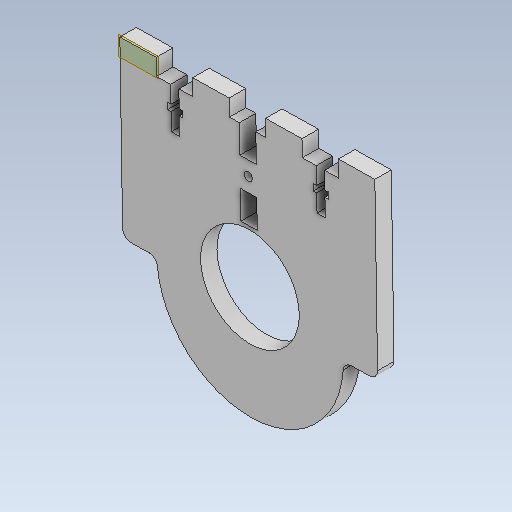
# Autodesk Inventor part: Деталь1
Saved by Autodesk Inventor 2021.1 (Build 251245010, 245A)
## iProperties
Created: 2023-03-16
Part Number: Деталь1
Material: Типовые
Document SubType Name: Modeling
Designer: User
Density: 1 g/cm^3
Appearance: По умолчанию
Author: User
Autodesk Inventor part; units mm, degrees
ref_plane "YZ Plane" through (0, 0, 0) normal (1, 0, 0) x (0, 1, 0)
ref_plane "XZ Plane" through (0, 0, 0) normal (0, 1, 0) x (-1, 0, 0)
ref_plane "XY Plane" through (0, 0, 0) normal (0, 0, 1) x (1, 0, 0)
ref_plane "РабПлоскость1" through (67.2056, 19.9956, 394.3851) normal (0, 0, -1) x (-0.9999, -0.0165, 0)
sketch "Эскиз1" plane through (67.2056, 19.9956, 394.3851) normal (0, 0, -1) x (-0.9999, -0.0165, 0)
  line L0 (-9.6218, -57.1442) -> (-3, -57.1442) projected
  arc A0 (-9.6218, -57.1442) -> (-12.6119, -59.9009) centre (-9.6218, -60.1442) ccw projected
  arc A1 (-3, -57.1442) -> (0, -54.1442) centre (-3, -54.1442) ccw projected
  line L1 (0, -54.1442) -> (0, 5.8558) projected
  line L2 (0, 5.8558) -> (-13.2857, 5.8558) projected
  line L3 (-13.2857, -0.1442) -> (-13.2857, 5.8558) projected
  line L4 (-13.2857, -0.1442) -> (-26.5714, -0.1442)
  line L5 (-26.5714, -0.1442) -> (-26.5714, 5.8558)
  line L6 (-26.5714, 5.8558) -> (-39.8571, 5.8558) projected
  line L7 (-39.8571, -0.1442) -> (-39.8571, 5.8558) projected
  line L8 (-39.8571, -0.1442) -> (-53.1429, -0.1442)
  line L9 (-53.1429, -0.1442) -> (-53.1429, 5.8558)
  line L10 (-53.1429, 5.8558) -> (-66.4286, 5.8558) projected
  line L11 (-66.4286, -0.1442) -> (-66.4286, 5.8558) projected
  line L12 (-66.4286, -0.1442) -> (-79.7143, -0.1442)
  line L13 (-79.7143, -0.1442) -> (-79.7143, 5.8558)
  line L14 (-79.7143, 5.8558) -> (-93, 5.8558) projected
  line L15 (-93, 5.8558) -> (-93, -54.1442) projected
  arc A2 (-93, -54.1442) -> (-90, -57.1442) centre (-90, -54.1442) ccw projected
  line L16 (-90, -57.1442) -> (-83.3782, -57.1442) projected
  arc A3 (-80.3881, -59.9009) -> (-83.3782, -57.1442) centre (-83.3782, -60.1442) ccw projected
  arc A4 (-80.3881, -59.9009) -> (-12.6119, -59.9009) centre (-46.5, -57.1442) ccw projected
  circle A5 centre (-46.5, -50.1442) radius 18
  line L17 (-74.5714, -0.1442) -> (-79.7143, -0.1442) projected
  line L18 (-21.4286, -0.1442) -> (-26.5714, -0.1442) projected
  line L19 (-49.5, -0.1442) -> (-53.1429, -0.1442) projected
  circle A6 centre (-46.5, -50.1442) radius 18 construction
  point P0 (67.5262, -18.8845)
  dimension "d0" = 6
  constraints: 12 end point, 1 centre point, 1 coincident, 1 concentric
  measures "d0" distance of L3.start L2.end
extrude "Выдавливание1" add sketch "Эскиз1" along normal blind 6
sketch "Эскиз2" plane through (67.2056, 19.9956, 388.3851) normal (0, 0, -1) x (-0.9999, -0.0165, 0)
  circle A0 centre (-46.5, -15.5) radius 1.5 projected
  line L0 (-49.5, -10.3334) -> (-49.5, -0.1442) construction
  line L1 (-43.5, -0.1442) -> (-43.5, -10.3334) construction
  line L2 (-43.5, -20.6667) -> (-43.5, -31) construction
  line L3 (-49.5, -31) -> (-49.5, -20.6667) construction
  line L4 (-49.5, -31) -> (-43.5, -31)
  line L5 (-43.5, -31) -> (-43.5, -20.6667)
  line L6 (-43.5, -20.6667) -> (-49.5, -20.6667)
  line L7 (-49.5, -20.6667) -> (-49.5, -31)
  line L8 (-49.5, -10.3334) -> (-43.5, -10.3334)
  line L9 (-43.5, -10.3334) -> (-43.5, -0.1442)
  line L10 (-43.5, -0.1442) -> (-49.5, -0.1442)
  line L11 (-49.5, -0.1442) -> (-49.5, -10.3334)
  line L12 (-17.1786, -8.65) -> (-17.1786, -6.35)
  line L13 (-17.1786, -6.35) -> (-18.4286, -6.35)
  line L14 (-18.4286, -6.35) -> (-18.4286, -0.1442)
  line L15 (-21.4286, -0.1442) -> (-21.4286, -6.35)
  line L16 (-21.4286, -6.35) -> (-22.6786, -6.35)
  line L17 (-22.6786, -6.35) -> (-22.6786, -8.65)
  line L18 (-22.6786, -8.65) -> (-21.4286, -8.65)
  line L19 (-21.4286, -8.65) -> (-21.4286, -15)
  line L20 (-21.4286, -15) -> (-18.4286, -15)
  line L21 (-18.4286, -15) -> (-18.4286, -8.65)
  line L22 (-18.4286, -8.65) -> (-17.1786, -8.65)
  line L23 (-21.4286, -0.1442) -> (-18.4286, -0.1442)
  line L24 (-46.5, -10.3334) -> (-46.5, -0.1442) construction
  line L25 (-75.8214, -8.65) -> (-75.8214, -6.35)
  line L26 (-75.8214, -6.35) -> (-74.5714, -6.35)
  line L27 (-74.5714, -6.35) -> (-74.5714, -0.1442)
  line L28 (-71.5714, -0.1442) -> (-71.5714, -6.35)
  line L29 (-71.5714, -6.35) -> (-70.3214, -6.35)
  line L30 (-70.3214, -6.35) -> (-70.3214, -8.65)
  line L31 (-70.3214, -8.65) -> (-71.5714, -8.65)
  line L32 (-71.5714, -8.65) -> (-71.5714, -15)
  line L33 (-71.5714, -15) -> (-74.5714, -15)
  line L34 (-74.5714, -15) -> (-74.5714, -8.65)
  line L35 (-74.5714, -8.65) -> (-75.8214, -8.65)
  line L36 (-71.5714, -0.1442) -> (-74.5714, -0.1442)
  point P0 (67.5262, -18.8845)
  constraints: 66 end point, 12 symmetric about line, 7 horizontal, 7 vertical, 4 parallel, 2 midpoint, 2 perpendicular, 12 other
extrude "Выдавливание2" cut sketch "Эскиз2" against normal blind 6
equation "\"d1\" = d0"
equation "\"d3\" = d0"
